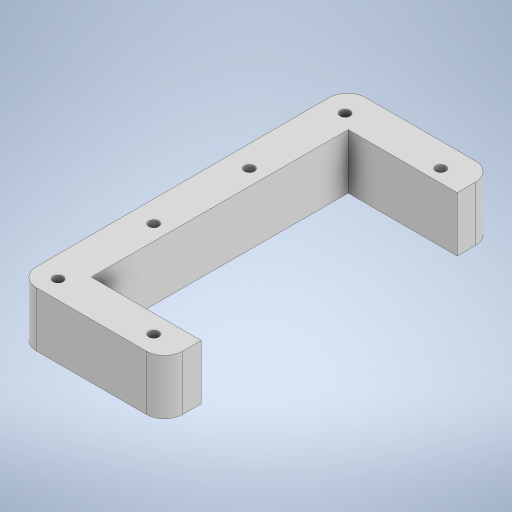
# Autodesk Inventor part: FINALBH
Saved by Autodesk Inventor 2024 (Build 280153000, 153)
## iProperties
Created: 2023-08-14
Part Number: FINALBH
Material: Generic
Document SubType Name: Modeling
Designer: s137416
Density: 1 g/cm^3
Appearance: Default
Author: s137416
Autodesk Inventor part; units mm, degrees
ref_plane "YZ Plane" through (0, 0, 0) normal (1, 0, 0) x (0, 1, 0)
ref_plane "XZ Plane" through (0, 0, 0) normal (0, 1, 0) x (-1, 0, 0)
ref_plane "XY Plane" through (0, 0, 0) normal (0, 0, 1) x (1, 0, 0)
sketch "Sketch1" plane through (0, 0, 0) normal (0, 1, 0) x (-1, 0, 0)
  line L0 (-50.8, 114.3) -> (50.8, 114.3)
  line L1 (50.8, 114.3) -> (50.8, -114.3)
  line L2 (50.8, -114.3) -> (-50.8, -114.3)
  line L3 (-50.8, -114.3) -> (-50.8, 114.3)
  line L4 (-50.8, 114.3) -> (50.8, -114.3) construction
  line L5 (50.8, 114.3) -> (-50.8, -114.3) construction
  line L6 (-50.8, 88.9) -> (25.4, 88.9)
  line L7 (25.4, 88.9) -> (24.8543, -88.9)
  line L8 (24.8543, -88.9) -> (-50.8, -88.9)
  point P0 (0, 0)
  dimension "d0" = 101.6
  dimension "d1" = 228.6
  dimension "d2" = 76.2
  dimension "d3" = 25.4
  dimension "d4" = 25.4
  constraints: 18 end point, 3 perpendicular, 2 midpoint, 2 parallel, 2 point on line, 1 horizontal
  measures "d0" distance of L1.end L2.end
  measures "d1" distance of L0.end L1.end
  measures "d2" distance of L6.start L6.end
  measures "d3" distance between parallel lines of L0 L6
  measures "d4" distance from line of L2 L7.end
extrude "Extrusion1" add sketch "Sketch1" along normal blind 38.1 contours L0 L1 L2 L3 L8 L7 L6
fillet "Fillet1" radius 12.7 4 edges at (50.8, 19.05, 114.3) (-50.8, 19.05, 114.3) (-50.8, 19.05, -114.3) (50.8, 19.05, -114.3)
sketch "Sketch2" plane through (0, 38.1, 0) normal (0, 1, 0) x (1, 0, 0)
  line L0 (-38.1, -114.3) -> (38.1, -114.3) projected
  circle A0 centre (-35.8052, -101.6) radius 3.3782
  line L1 (-35.8052, -101.6) -> (-35.8052, 101.6) construction
  line L2 (-35.8052, -101.6) -> (40.3948, -101.6) construction
  line L3 (-35.8052, 101.6) -> (40.3948, 101.6) construction
  circle A1 centre (-35.8052, -88.3158) radius 3.3782 construction
  line L4 (-39.1834, -98.2218) -> (-30.0963, -98.2218) construction
  circle A2 centre (-35.8052, -75.0316) radius 3.3782 construction
  circle A3 centre (-35.8052, -61.7474) radius 3.3782 construction
  circle A4 centre (-35.8052, -48.4632) radius 3.3782 construction
  circle A5 centre (-35.8052, -35.179) radius 3.3782 construction
  circle A6 centre (-35.8052, -21.8948) radius 3.3782 construction
  circle A7 centre (-35.8052, -8.6106) radius 3.3782 construction
  circle A8 centre (-35.8052, 4.6736) radius 3.3782 construction
  circle A9 centre (-35.8052, 17.9578) radius 3.3782 construction
  circle A10 centre (-35.8052, 31.242) radius 3.3782 construction
  circle A11 centre (-35.8052, 44.5262) radius 3.3782 construction
  circle A12 centre (-35.8052, 57.8104) radius 3.3782 construction
  circle A13 centre (-35.8052, 71.0946) radius 3.3782 construction
  circle A14 centre (-35.8052, 84.3788) radius 3.3782 construction
  circle A15 centre (-35.8052, 97.663) radius 3.3782 construction
  circle A16 centre (-22.521, -101.6) radius 3.3782 construction
  circle A17 centre (-9.2368, -101.6) radius 3.3782 construction
  circle A18 centre (4.0474, -101.6) radius 3.3782 construction
  circle A19 centre (17.3316, -101.6) radius 3.3782 construction
  circle A20 centre (30.6158, -101.6) radius 3.3782 construction
  circle A21 centre (43.9, -101.6) radius 3.3782 construction
  circle A22 centre (30.6158, 97.663) radius 3.3782 construction
  circle A23 centre (30.6158, -101.6) radius 3.3782 construction
  circle A24 centre (-35.8052, 97.663) radius 3.3782 construction
  circle A25 centre (-35.8052, 31.242) radius 3.3782 construction
  circle A26 centre (-35.8052, -35.179) radius 3.3782 construction
  circle A27 centre (-35.8052, -35.179) radius 3.3782
  circle A28 centre (-35.8052, 31.242) radius 3.3782
  circle A29 centre (-35.8052, 97.663) radius 3.3782
  circle A30 centre (30.6158, 97.663) radius 3.3782
  circle A31 centre (30.6158, -101.6) radius 3.3782
  point P0 (0, 0)
  point P1 (-35.8052, -25.4)
  point P2 (-35.8052, 25.4)
  dimension "d8" = 12.7
  dimension "d9" = 76.2
  dimension "d10" = 127
  dimension "d11" = 203.2
  dimension "d12" = 76.2
  dimension "d13" = 6.7564
  dimension "d22" = 13.2842
  dimension "d25" = 13.2842
  dimension "d30" = 13.2842
  dimension "d33" = 13.2842
  dimension "d38" = 6.7564
  dimension "d39" = 6.7564
  dimension "d40" = 6.7564
  dimension "d41" = 6.7564
  dimension "d42" = 6.7564
  dimension "d43" = 6.7564
  dimension "d44" = 6.7564
  dimension "d45" = 6.7564
  dimension "d46" = 6.7564
  constraints: 32 centre point, 13 coincident, 8 end point, 4 horizontal, 3 equal radius, 2 point on line, 2 vertical, 1 horizontal alignment, 1 tangent, 38 other
  measures "d8" distance from line of L0 point (-35.805, -101.6)
  measures "d9" distance of point (-35.805, -25.4) point (-35.805, -101.6)
  measures "d10" distance of point (-35.805, 25.4) point (-35.805, -101.6)
  measures "d11" distance of point (-35.805, 101.6) point (-35.805, -101.6)
  measures "d12" distance of point (40.395, -101.6) point (-35.805, -101.6)
  measures "d13" diameter of A0
  measures "d22" distance of A1.centre L1.start
  measures "d25" distance of A1.centre A2.centre
  measures "d30" distance of A16.centre L1.start
  measures "d33" distance of A16.centre A17.centre
  measures "d38" diameter of A22
  measures "d39" diameter of A23
  measures "d40" diameter of A24
  measures "d41" diameter of A25
  measures "d42" diameter of A26
  measures "d43" diameter of A28
  measures "d44" diameter of A29
  measures "d45" diameter of A30
  measures "d46" diameter of A31
extrude "Extrusion4" cut sketch "Sketch2" against normal through all
equation "\"d25\" = d22"
equation "\"d30\" = d22"
equation "\"d33\" = d22"
body "Solid1"
